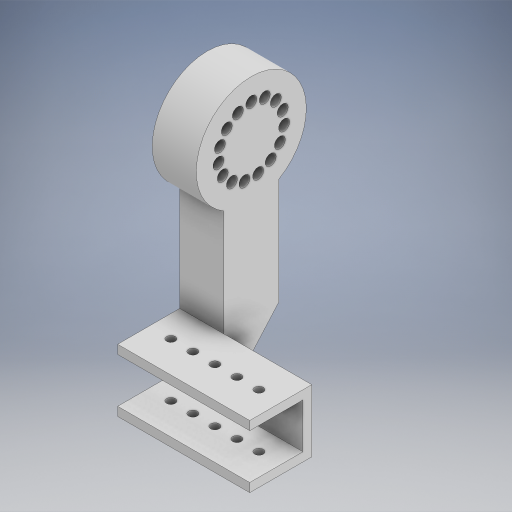
# Autodesk Inventor part: 2024-900-004-REV2
Saved by Autodesk Inventor 2024.2 (Build 282272000, 272)
## iProperties
Created: 2024-03-11
Part Number: 2024-900-004-REV2
Material: Generic
Document SubType Name: Modeling
Designer: rohan
Density: 1 g/cm^3
Appearance: Default
Author: rohan
Autodesk Inventor part; units mm, degrees
ref_plane "YZ Plane" through (0, 0, 0) normal (1, 0, 0) x (0, 1, 0)
ref_plane "XZ Plane" through (0, 0, 0) normal (0, 1, 0) x (-1, 0, 0)
ref_plane "XY Plane" through (0, 0, 0) normal (0, 0, 1) x (1, 0, 0)
sketch "Sketch1" plane through (0, 0, 0) normal (1, 0, 0) x (0, 1, 0)
  line L0 (12.954, 12.7) -> (12.954, -12.954)
  line L1 (12.954, -12.954) -> (-12.954, -12.954)
  line L2 (-12.954, -12.954) -> (-12.954, 12.7)
  line L3 (12.954, 17.78) -> (18.034, 17.78)
  line L4 (18.034, 17.78) -> (18.034, -18.034)
  line L5 (18.034, -18.034) -> (-18.034, -18.034)
  line L6 (-18.034, -18.034) -> (-18.034, 17.78)
  line L7 (-18.034, 17.78) -> (-12.954, 17.78)
  line L8 (12.954, 12.7) -> (12.954, 17.78)
  line L9 (-12.954, 12.7) -> (-12.954, 17.78)
  point P0 (0, 0)
  constraints: 20 end point, 2 parallel, 2 perpendicular, 2 other
extrude "Extrusion1" add sketch "Sketch1" along normal blind 76.2
sketch "Sketch3" plane through (76.2, 18.034, 17.78) normal (0, 1, 0) x (1, 0, 0)
  circle A0 centre (-12.7, 18.034) radius 2.4892
  line L0 (-76.2, 35.814) -> (0, 35.814) projected
  line L1 (0, 0) -> (0, 30.734) projected
  circle A1 centre (-25.4, 18.034) radius 2.4892
  circle A2 centre (-38.1, 18.034) radius 2.4892
  circle A3 centre (-50.8, 18.034) radius 2.4892
  circle A4 centre (-63.5, 18.034) radius 2.4892
  point P0 (-76.2, 17.78)
  point P1 (-63.5, 35.814)
  dimension "d11" = 4.9784
  dimension "d13" = 12.7
  dimension "d14" = 12.7
  dimension "d17" = 12.7
  dimension "d36" = 4.9784
  dimension "d37" = 12.7
  constraints: 5 centre point, 1 horizontal, 6 other
  measures "d11" diameter of A0
  measures "d13" distance from line of A0.centre L1
  measures "d14" horizontal distance of L1.end A0.centre
  measures "d17" distance of A0.centre A1.centre
  measures "d36" diameter of A4
  measures "d37" distance of A3.centre A4.centre
extrude "Extrusion6" cut sketch "Sketch3" against normal blind 66.675
sketch "Sketch6" plane through (0, 0, 0) normal (-1, 0, 0) x (0, 0, 1)
  line L0 (-18.034, 18.034) -> (17.78, 18.034) projected
  line L1 (-18.034, 18.034) -> (-49.784, 18.034)
  line L2 (17.78, -18.034) -> (-18.034, -18.034) projected
  line L3 (-49.784, 18.034) -> (-18.034, -18.034)
  line L4 (-18.034, -18.034) -> (-18.034, 18.034) projected
  point P0 (0, 0)
  dimension "d40" = 31.75
  constraints: 4 end point, 1 horizontal
  measures "d40" distance of L0.start L1.end
extrude "Extrusion7" add sketch "Sketch6" against normal blind 25.4
sketch "Sketch7" plane through (0, 18.034, 17.78) normal (0, 1, 0) x (1, 0, 0)
  circle A0 centre (38.1, 18.034) radius 2.4892 projected
  circle A1 centre (50.8, 18.034) radius 2.4892 projected
  circle A2 centre (25.4, 18.034) radius 2.4892 projected
  circle A3 centre (63.5, 18.034) radius 2.4892 projected
  circle A4 centre (12.7, 18.034) radius 2.4892 projected
  line L0 (0, 0) -> (0, 67.564) projected
  line L1 (0, 0) -> (76.2, 0) projected
  line L2 (76.2, 35.814) -> (76.2, 0) projected
  line L3 (25.4, 35.814) -> (76.2, 35.814) projected
  line L4 (25.4, 67.564) -> (25.4, 35.814) projected
  line L5 (0, 67.564) -> (25.4, 67.564) projected
  line L6 (0, 35.814) -> (25.4, 35.814) projected
  line L7 (25.4, 35.814) -> (0, 35.814)
  point P0 (0, 17.78)
  constraints: 2 end point, 1 collinear
extrude "Extrusion8" add sketch "Sketch7" along normal blind 88.9 contours L0 L5 L4 L6
sketch "Sketch8" plane through (25.4, 0, 0) normal (1, 0, 0) x (0, 0, -1)
  line L0 (18.034, -18.034) -> (18.034, 18.034) projected
  line L1 (18.034, -18.034) -> (49.784, 18.034) projected
  line L2 (49.784, 18.034) -> (49.784, 106.934) projected
  line L3 (18.034, 106.934) -> (49.784, 106.934) projected
  line L4 (18.034, 18.034) -> (18.034, 106.934) projected
  line L5 (49.784, 106.934) -> (18.034, 106.934) projected
  circle A0 centre (33.909, 106.934) radius 31.75
  point P0 (0, 0)
  dimension "d45" = 63.5
  constraints: 1 centre point, 1 midpoint
  measures "d45" diameter of A0
extrude "Extrusion9" add sketch "Sketch8" against normal up to surface (25.4 mm away) contours A0 L2 L3 L4 | L4 L3 L2 A0
sketch "Sketch9" plane through (25.4, 0, 0) normal (1, 0, 0) x (0, 0, -1)
  line L0 (18.034, 18.034) -> (18.034, 79.4377) projected
  line L1 (18.034, -18.034) -> (18.034, 18.034) projected
  line L2 (18.034, -18.034) -> (49.784, 18.034) projected
  line L3 (49.784, 18.034) -> (49.784, 79.4377) projected
  arc A0 (49.784, 79.4377) -> (18.034, 79.4377) centre (33.909, 106.934) ccw projected
  circle A1 centre (33.909, 106.934) radius 19.05
  circle A2 centre (33.909, 125.984) radius 3.175
  circle A3 centre (26.1607, 124.337) radius 3.175
  circle A4 centre (19.7521, 119.6809) radius 3.175
  circle A5 centre (15.7914, 112.8208) radius 3.175
  circle A6 centre (14.9634, 104.9427) radius 3.175
  circle A7 centre (17.4112, 97.409) radius 3.175
  circle A8 centre (22.7117, 91.5222) radius 3.175
  circle A9 centre (29.9483, 88.3003) radius 3.175
  circle A10 centre (37.8697, 88.3003) radius 3.175
  circle A11 centre (45.1063, 91.5222) radius 3.175
  circle A12 centre (50.4068, 97.409) radius 3.175
  circle A13 centre (52.8546, 104.9427) radius 3.175
  circle A14 centre (52.0266, 112.8208) radius 3.175
  circle A15 centre (48.0659, 119.6809) radius 3.175
  circle A16 centre (41.6573, 124.337) radius 3.175
  point P0 (0, 0)
  dimension "d48" = 38.1
  dimension "d49" = 6.35
  dimension "d52" = 360
  constraints: 15 centre point, 1 coincident, 1 vertical alignment, 33 other
  measures "d49" diameter of A2
extrude "Extrusion10" cut sketch "Sketch9" against normal blind 25.4 contours A1 A13 | A1 A13 | A14 A1 | A1 A14 | A12 A1 | A1 A12 | A15 A1 | A1 A15 | A11 A1 | A1 A11 | A16 A1 | A1 A16 | A10 A1 | A1 A10 | A2 A1 | A1 A2 | A9 A1 | A1 A9 | A3 A1 | A1 A3 | A8 A1 | A1 A8 | A4 A1 | A1 A4 | A7 A1 | A1 A7 | A5 A1 | A1 A5 | A6 A1 | A1 A6
body "Solid1"
